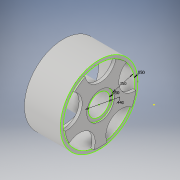
# Autodesk Inventor part: wheal
Saved by Autodesk Inventor 2017 SP1 (Build 210196100, 196)
## iProperties
Created: 2016-12-04
Part Number: wheal
Material: Generic
Document SubType Name: Modeling
Designer: rbibb
Density: 1 g/cm^3
Appearance: Default
Author: rbibb
Autodesk Inventor part; units mm, degrees
ref_plane "YZ Plane" through (0, 0, 0) normal (1, 0, 0) x (0, 1, 0)
ref_plane "XZ Plane" through (0, 0, 0) normal (0, 1, 0) x (-1, 0, 0)
ref_plane "XY Plane" through (0, 0, 0) normal (0, 0, 1) x (1, 0, 0)
sketch "Sketch1" plane through (0, 0, 0) normal (1, 0, 0) x (0, 1, 0)
  circle A0 centre (11.1737, 22.3473) radius 5.588
  circle A1 centre (11.1737, 22.3473) radius 4.318
  circle A2 centre (11.1737, 22.3473) radius 14.478
  circle A3 centre (11.1737, 22.3473) radius 15.748
  point P0 (0, 0)
  dimension "d0" = 11.176
  dimension "d1" = 1.27
  dimension "d2" = 1.27
  dimension "d3" = 8.89
  constraints: 4 centre point
  measures "d0" diameter of A0
  measures "d1" radial gap between concentric circles of A0 A1
  measures "d2" radial gap between concentric circles of A3 A2
  measures "d3" radial gap between concentric circles of A2 A0
extrude "Extrusion1" add sketch "Sketch1" against normal blind 14.478 contours A3
extrude "Extrusion2" add sketch "Sketch1" against normal blind 14.478 contours A0
sketch "Sketch2" plane through (0, 11.1737, 22.3473) normal (1, 0, 0) x (0, 0, -1)
  circle A0 centre (0, 0) radius 14.478 projected
  circle A1 centre (0, 0) radius 15.748 projected
  circle A2 centre (0, 0) radius 5.588 projected
  circle A3 centre (0, 0) radius 4.318 projected
  point P0 (22.3473, -11.1737)
extrude "Extrusion3" add sketch "Sketch2" along normal mid plane 1.27 contours A0
sketch "Sketch3" plane through (0.635, 11.1737, 22.3473) normal (1, 0, 0) x (0, 0, -1)
  circle A0 centre (0, 0) radius 14.478 projected
  arc A1 (-6.1954, 13.0855) -> (6.1954, 13.0855) centre (0, 14.478) ccw
  arc A2 (6.1954, 13.0855) -> (-6.1954, 13.0855) centre (0, 0) ccw
  arc A3 (-14.3595, -1.8486) -> (-10.5305, 9.9358) centre (-13.7694, 4.4739) ccw
  arc A4 (-10.5305, 9.9358) -> (-14.3595, -1.8486) centre (0, 0) ccw
  arc A5 (-2.6792, -14.2279) -> (-12.7036, -6.9448) centre (-8.51, -11.7129) ccw
  arc A6 (-12.7036, -6.9448) -> (-2.6792, -14.2279) centre (0, 0) ccw
  arc A7 (12.7036, -6.9448) -> (2.6792, -14.2279) centre (8.51, -11.7129) ccw
  arc A8 (2.6792, -14.2279) -> (12.7036, -6.9448) centre (0, 0) ccw
  arc A9 (10.5305, 9.9358) -> (14.3595, -1.8486) centre (13.7694, 4.4739) ccw
  arc A10 (14.3595, -1.8486) -> (10.5305, 9.9358) centre (0, 0) ccw
  point P0 (22.3473, -11.1737)
  dimension "d10" = 12.7
  dimension "d13" = 360
  constraints: 25 point on circle, 10 centre point, 1 coincident, 1 vertical alignment, 32 other
  measures "d10" diameter of A1
extrude "Extrusion4" cut sketch "Sketch3" against normal up to next contours A0 A9 | A1 A0 | A0 A7 | A3 A0 | A0 A5
body "Solid1"
